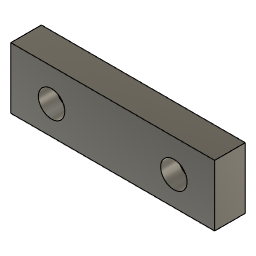
5tormachViseJaws (Autodesk Fusion 360 design; units mm, degrees)
Autodesk Fusion 360 part; units mm, degrees
sketch "Sketch1" plane through (0, 0, 0) normal (0, 1, 0) x (1, 0, 0) in component "softJaws"
  line L0 (0, -38.1) -> (127, -38.1)
  line L1 (127, -38.1) -> (127, 0)
  line L2 (127, 0) -> (0, 0)
  line L3 (0, 0) -> (0, -38.1)
  dimension "d1" = 127
  dimension "d2" = 38.1
  constraint horizontal L0
  constraint vertical L1
  constraint horizontal L2
  constraint vertical L3
  constraint coincident L2.end L3.start
  measures "d1" distance of L0.start L0.end
  measures "d2" distance of L0.start L2.end
extrude "Extrude1" add sketch "Sketch1" along normal blind 19.05 in component "softJaws"
sketch "Sketch2" plane through (0, 0, 0) normal (0, -1, 0) x (1, 0, 0) in component "softJaws"
  line L0 (0, 38.1) -> (0, 0)
  line L1 (0, 0) -> (127, 0)
  line L2 (127, 0) -> (127, 38.1)
  line L3 (127, 38.1) -> (0, 38.1)
  circle A0 centre (25.4, 17.78) radius 6.35
  circle A1 centre (101.6, 17.78) radius 6.35
  dimension "d11" = 12.7
  dimension "d12" = 12.7
  dimension "d13" = 76.2
  dimension "d14" = 17.78
  dimension "d15" = 17.78
  dimension "d16" = 25.4
  measures "d11" diameter of A0
  measures "d12" diameter of A1
  measures "d13" distance of A0.centre A1.centre
  measures "d14" distance of L1 A0.centre
  measures "d15" distance of L1 A1.centre
  measures "d16" distance of L2 A1.centre
extrude "Extrude2" cut sketch "Sketch2" against normal through all contours A0 | A1 in component "softJaws"
sketch "Sketch3" plane through (0, 0, 0) normal (0, -1, 0) x (1, 0, 0) in component "softJaws"
  circle A0 centre (101.6, 17.78) radius 6.35
  circle A1 centre (25.4, 17.78) radius 6.35
  line L0 (0, 38.1) -> (0, 0)
  line L1 (0, 0) -> (127, 0)
  line L2 (127, 0) -> (127, 38.1)
  line L3 (127, 38.1) -> (0, 38.1)
  circle A2 centre (25.4, 17.78) radius 8.255
  circle A3 centre (101.6, 17.78) radius 8.255
  dimension "d18" = 16.51
  dimension "d19" = 16.51
  constraint concentric A1 A2
  constraint concentric A0 A3
  measures "d18" diameter of A2
  measures "d19" diameter of A3
extrude "Extrude3" cut sketch "Sketch3" against normal blind 11.176 contours A2 | A3 in component "softJaws"
component "softJaws" placed x (1, 0, 0) y (0, 1, 0) z (0, 0, 1) at (0, 0, 0)
equation "d1 = length"
equation "d2 = height"
equation "d3 = thickness"
equation "length = 5 in"
equation "height = 1.5 in"
equation "thickness = 0.75 in"
equation "holeDiameter = 0.5 in"
equation "holeDistance = 3 in"
equation "holeVise = 0.7 in"
equation "d11 = holeDiameter"
equation "d12 = holeDiameter"
equation "d13 = holeDistance"
equation "d14 = holeVise"
equation "d15 = holeVise"
equation "d16 = ( length - holeDistance ) / 2"
